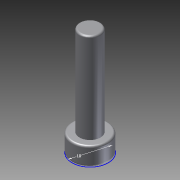
# Autodesk Inventor part: pern frontissa
Saved by Autodesk Inventor 2012 SP1 (Build 160190100, 190)
## iProperties
Created: 2015-03-29
Part Number: pern frontissa
Material: Default
Document SubType Name: Modeling
Designer: sheina
Density: 1 g/cm^3
Author: sheina
Autodesk Inventor part; units mm, degrees
ref_plane "YZ Plane" through (0, 0, 0) normal (1, 0, 0) x (0, 1, 0)
ref_plane "XZ Plane" through (0, 0, 0) normal (0, 1, 0) x (-1, 0, 0)
ref_plane "XY Plane" through (0, 0, 0) normal (0, 0, 1) x (1, 0, 0)
sketch "Boceto1" plane through (0, 0, 0) normal (0, 0, 1) x (1, 0, 0)
  circle A0 centre (0, 0) radius 5
  dimension "d0" = 10
  constraints: 1 centre point, 1 coincident
  measures "d0" diameter of A0
extrude "Extrusión1" add sketch "Boceto1" along normal blind 30
sketch "Boceto2" plane through (0, 0, 30) normal (0, 0, 1) x (1, 0, 0)
  circle A0 centre (0, 0) radius 5 projected
  circle A1 centre (0, 0) radius 2.9
  dimension "d3" = 5.8
  constraints: 1 centre point, 1 coincident
  measures "d3" diameter of A1
extrude "Extrusión2" cut sketch "Boceto2" against normal blind 25
fillet "Empalme1" radius 0.5 3 edges at (-2.9, 0, 30) (-5, 0, 5) (-5, 0, 0)
